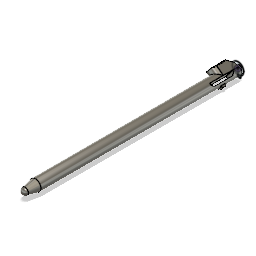
Nintendo 2DS Stylus v2 (Autodesk Fusion 360 design; units mm, degrees)
Autodesk Fusion 360 part; units mm, degrees
sketch "Sketch1" plane through (0, 0, 0) normal (0, 0, 1) x (1, 0, 0)
  circle A0 centre (0, 0) radius 2.45
  dimension "d1" = 4.9
  constraint coincident A0.centre origin
  measures "d1" diameter of A0
extrude "Extrude1" add sketch "Sketch1" along normal blind 94
sketch "Sketch2" plane through (0, 0, 0) normal (1, 0, 0) x (0, 0, -1)
  line L0 (0, 0) -> (0, -2.45)
  line L1 (0, -2.45) -> (-1, -2.45)
  line L2 (0, -2.45) -> (-3.2, -2.45)
  line L3 (-3.2, -2.45) -> (-3.2, 3.95)
  line L4 (-3.2, 3.95) -> (0, 3.95)
  line L5 (0, 3.95) -> (0, -2.45)
  line L6 (0, -2.45) -> (0, 1.95)
  line L7 (0, 1.95) -> (-1, 1.95)
  line L8 (0, -2.45) -> (-1, 1.95)
  line L9 (-1, 1.95) -> (-3.2, 3.95)
  line L10 (0, 0) -> (-3.2, 0)
  line L11 (-3.2, 3.95) -> (-10.3, 3.95)
  line L12 (-10.3, 3.95) -> (-3.2, 3.95)
  line L13 (-3.2, 3.95) -> (-3.2, 0)
  line L14 (-3.2, 0) -> (-10.3, 0)
  line L15 (-10.3, 0) -> (-10.3, 3.95)
  dimension "d4" = 2.45
  dimension "d5" = 1
  dimension "d8" = 3.2
  dimension "d9" = 6.4
  dimension "d10" = 4.4
  dimension "d11" = 1
  dimension "d14" = 7.1
  constraint coincident L0.start L10.start
  constraint vertical L0
  constraint horizontal L1
  constraint horizontal L2
  constraint vertical L3
  constraint horizontal L4
  constraint vertical L5
  constraint perpendicular L1 L6
  constraint perpendicular L6 L7
  constraint coincident L3 L10.end
  constraint perpendicular L3 L10
  constraint perpendicular L3 L11
  constraint horizontal L12
  constraint vertical L13
  constraint horizontal L14
  constraint vertical L15
  measures "d4" distance of L0.start L0.end
  measures "d5" distance of L0.end L1.end
  measures "d8" distance of L0.end L2.end
  measures "d9" distance of L0.end L4.end
  measures "d10" distance of L0.end L6.end
  measures "d11" distance of L6.end L7.end
  measures "d14" distance of L3.end L11.end
extrude "Extrude3" add sketch "Sketch2" along normal mid plane 4.9 contours L3 L8 L9 L10 L13 | L3 L11 L12 L13 L14 L15
extrude "Extrude2" cut sketch "Sketch2" along normal mid plane 12 contours L5 L6 L7 L8 L10 | L0 L5 L6 L8 L10 | L4 L5 L7 L9
sketch "Sketch3" plane through (0, 3.95, 0) normal (0, 1, 0) x (-1, 0, 0)
  line L0 (2.45, 10.3) -> (-2.45, 10.3)
  line L1 (-2.45, 10.3) -> (-2.45, 3.2)
  line L2 (-2.45, 3.2) -> (2.45, 3.2)
  line L3 (2.45, 3.2) -> (2.45, 10.3)
  circle A0 centre (0, 7.85) radius 2.45
  dimension "d17" = 4.9
  measures "d17" diameter of A0
extrude "Extrude4" cut sketch "Sketch3" against normal blind 4.1 contours L0 L3 A0 | L0 L1 A0
extrude "Extrude5" add 2 faces at (0.1162, 1.575, 10.3) (-0.1207, 1.5744, 10.3) along direction (0, 0, -1) blind 3.8
sketch "Sketch4" plane through (2.45, 0, 0) normal (1, 0, 0) x (0, 0, -1)
  line L0 (-7.85, 3.95) -> (-7.85, 0)
  line L1 (-7.85, 0) -> (-0.5568, 0)
  line L2 (-0.5568, 0) -> (-1, 1.95)
  line L3 (-1, 1.95) -> (-3.2, 3.95)
  line L4 (-3.2, 3.95) -> (-7.85, 3.95)
  line L5 (-3.2, 3.95) -> (-10.3, 3.95)
  line L6 (-10.3, 3.95) -> (-9.05, 3.95)
  line L7 (-9.05, 3.95) -> (-8.3, 3.95)
  line L8 (-8.3, 3.95) -> (-8.05, 3.95)
  line L9 (-8.05, 3.95) -> (-7.3, 3.95)
  line L10 (-7.3, 3.95) -> (-7.05, 3.95)
  line L11 (-7.05, 3.95) -> (-6.3, 3.95)
  line L12 (-6.3, 3.95) -> (-6.05, 3.95)
  line L13 (-6.05, 3.95) -> (-5.3, 3.95)
  line L14 (-8.675, 3.95) -> (-8.675, 3.45)
  line L15 (-9.05, 3.95) -> (-8.675, 3.45)
  line L16 (-8.675, 3.45) -> (-8.3, 3.95)
  line L17 (-7.675, 3.95) -> (-7.675, 3.45)
  line L18 (-6.675, 3.95) -> (-6.675, 3.45)
  line L19 (-5.675, 3.95) -> (-5.675, 3.45)
  line L20 (-8.05, 3.95) -> (-7.675, 3.45)
  line L21 (-7.675, 3.45) -> (-7.3, 3.95)
  line L22 (-7.05, 3.95) -> (-6.675, 3.45)
  line L23 (-6.3, 3.95) -> (-6.675, 3.45)
  line L24 (-6.05, 3.95) -> (-5.675, 3.45)
  line L25 (-5.675, 3.45) -> (-5.3, 3.95)
  line L26 (-5.3, 3.95) -> (-5.05, 3.95)
  line L27 (-5.05, 3.95) -> (-4.3, 3.95)
  line L28 (-4.675, 3.95) -> (-4.675, 3.45)
  line L29 (-5.05, 3.95) -> (-4.675, 3.45)
  line L30 (-4.675, 3.45) -> (-4.3, 3.95)
  dimension "d22" = 7.1
  dimension "d23" = 1.25
  dimension "d24" = 0.75
  dimension "d25" = 0.25
  dimension "d26" = 0.75
  dimension "d27" = 0.25
  dimension "d28" = 0.75
  dimension "d29" = 0.25
  dimension "d30" = 0.75
  dimension "d31" = 0.5
  dimension "d32" = 0.5
  dimension "d33" = 0.5
  dimension "d34" = 0.5
  dimension "d35" = 0.25
  dimension "d36" = 0.75
  dimension "d37" = 0.5
  constraint coincident L3.end L4.start
  constraint perpendicular L0 L5
  constraint parallel L5 L6
  constraint parallel L5 L7
  constraint parallel L5 L8
  constraint perpendicular L0 L9
  constraint parallel L4 L10
  constraint parallel L5 L11
  constraint parallel L5 L12
  constraint parallel L5 L13
  constraint midpoint L7 L14.start
  constraint perpendicular L7 L14
  constraint midpoint L9 L17.start
  constraint perpendicular L5 L17
  constraint midpoint L11 L18.start
  constraint perpendicular L5 L18
  constraint midpoint L13 L19.start
  constraint perpendicular L13 L19
  constraint coincident L4 L26.end
  constraint parallel L5 L27
  constraint midpoint L27 L28.start
  constraint perpendicular L5 L28
  measures "d22" distance of L3.end L5.end
  measures "d23" distance of L5.end L6.end
  measures "d24" distance of L6.end L7.end
  measures "d25" distance of L7.end L8.end
  measures "d26" distance of L8.end L9.end
  measures "d27" distance of L9.end L10.end
  measures "d28" distance of L10.end L11.end
  measures "d29" distance of L11.end L12.end
  measures "d30" distance of L12.end L13.end
  measures "d31" distance of L14.start L14.end
  measures "d32" distance of L17.start L17.end
  measures "d33" distance of L18.start L18.end
  measures "d34" distance of L19.start L19.end
  measures "d35" distance of L13.end L26.end
  measures "d36" distance of L26.end L27.end
  measures "d37" distance of L28.start L28.end
extrude "Extrude6" cut sketch "Sketch4" against normal blind 8.9 contours L0 L4 L5 L9 L17 L20 | L0 L5 L9 L20 | L4 L5 L9 L17 L21 | L4 L5 L11 L18 L22 | L4 L5 L11 L18 L23 | L4 L5 L27 L28 L30 | L4 L5 L13 L19 L24 | L4 L5 L27 L28 L29 | L4 L5 L13 L19 L25 | L5 L7 L14 L16 | L5 L7 L14 L15
sketch "Sketch5" plane through (0, 0, 0) normal (1, 0, 0) x (0, 0, -1)
  line L0 (0, 0) -> (0, -2.45)
  line L1 (0, -2.45) -> (-9.8, -2.45)
  line L2 (-9.8, -2.45) -> (-7.8, -2.45)
  ellipse E0 centre (-8.8, -2.45) end of major axis (-7.8, -2.45) minor radius 0.625
  line L3 (-9.8, -2.45) -> (-7.8, -2.45) construction
  line L4 (-8.8, -3.075) -> (-8.8, -1.825) construction
  line L5 (0, 0) -> (-8.8, 0)
  line L6 (-8.8, -2.45) -> (-8.8, -1.45)
  line L7 (-8.8, 0) -> (-3.8, 0)
  line L8 (-3.8, 1.45) -> (-13.8, 1.45)
  line L9 (-13.8, -1.45) -> (-3.8, -1.45)
  line L10 (-3.8, 0) -> (-13.8, 0) construction
  line L11 (-8.8, 0) -> (-15.25, 0)
  line L12 (-5.25, 1.45) -> (-12.35, 1.45)
  arc A0 (-12.35, 1.45) -> (-12.35, -1.45) centre (-12.35, 0) ccw
  line L13 (-12.35, -1.45) -> (-5.25, -1.45)
  arc A1 (-5.25, -1.45) -> (-5.25, 1.45) centre (-5.25, 0) ccw
  line L14 (-3.8, 0) -> (-13.8, 0) construction
  dimension "d40" = 2.45
  dimension "d41" = 9.8
  dimension "d42" = 2
  dimension "d43" = 1.25
  dimension "d44" = 1
  dimension "d45" = 5
  constraint coincident L0.start L5.start
  constraint vertical L0
  constraint perpendicular L0 L1
  constraint parallel L1 L2
  constraint midpoint L2 E0.centre
  constraint coincident L1.end E0
  constraint coincident E0 L4.start
  constraint coincident E0 L4.end
  constraint perpendicular L4 L5
  constraint coincident E0.centre L6.start
  constraint perpendicular L3 L6
  constraint parallel L5 L7
  constraint parallel L8 L9
  constraint parallel L5 L10
  constraint coincident L7.end L10.start
  constraint tangent L12 A0
  constraint tangent A0 L13
  constraint parallel L12 L13
  constraint tangent L13 A1
  constraint tangent L12 A1
  constraint midpoint A1 L7.end
  constraint midpoint A0 L10.end
  constraint coincident L10.end L14.end
  constraint parallel L11 L14
  measures "d40" distance of L0.start L0.end
  measures "d41" distance of L0.end L1.end
  measures "d42" distance of L1.end L2.end
  measures "d44" distance of E0.centre L6.end
  measures "d45" distance of L5.end L7.end
extrude "Extrude7" cut sketch "Sketch5" along normal mid plane 11 contours L5 L7 L9 L11 A0 L13 A1
extrude "Extrude8" add sketch "Sketch5" along normal mid plane 2 contours L1 L2 E0 | L1 L2 E0 L6 | L1 L2 E0 L6
sketch "Sketch6" plane through (0, 0, 94) normal (0, 0, 1) x (1, 0, 0)
  circle A0 centre (0, 0) radius 2.45
  circle A1 centre (0, 0) radius 1.5
  dimension "d50" = 3
  constraint coincident A0.centre A1.centre
  measures "d50" diameter of A1
extrude "Extrude9" cut sketch "Sketch6" against normal blind 6
fillet "Fillet1" radius 1.5 1 edges at (-1.3985, -0.5424, 94)
chamfer "Chamfer1" distance 4.5 distance2 0.95 1 edges at (-1.3985, -0.5424, 88) measured on face at (1.4981, -0.0748, 89.5)
move_face "OffsetFaces1" offset -0.5 2 faces at (0.8167, 0.65, 0.7045) (-0.8167, 2.6167, 1.7333)
sketch "Sketch7" plane through (0, 0, 0) normal (0, 0, 1) x (1, 0, 0)
  circle A0 centre (0, 0) radius 2.45
  line L0 (0, 0) -> (0, -3.075)
  line L1 (0, -3.075) -> (1, -3.075)
  line L2 (1, -3.075) -> (1, -2.2366)
  line L3 (1, -2.2366) -> (0, -2.2366)
  line L4 (0, -2.2366) -> (0, -3.075)
  line L5 (1, -3.075) -> (0.75, -3.075)
  line L6 (0.75, -3.075) -> (1.9563, -1.4749)
  dimension "d57" = 4.9
  dimension "d58" = 3.075
  dimension "d59" = 1
  dimension "d60" = 0.25
  constraint coincident A0.centre L0.start
  constraint vertical L0
  constraint horizontal L1
  constraint vertical L2
  constraint horizontal L3
  constraint vertical L4
  constraint coincident A0 L2.end
  constraint perpendicular L2 L5
  constraint coincident A0 L6.end
  constraint tangent A0 L6
  measures "d57" diameter of A0
  measures "d58" distance of A0.centre L0.end
  measures "d59" distance of L0.end L1.end
  measures "d60" distance of L1.end L5.end
move_body "Move1" bodies 1 to x (0.601815, 0.798636, 0) y (-0.798636, 0.601815, 0) z (0, 0, 1) at (0, 0, 0)
equation "d4 = ( 4.9 / 2 ) * 1 mm"
equation "d15 = ( 4.9 / 2 ) * 1 mm"
equation "d40 = ( 4.9 / 2 ) * 1 mm"
equation "d56 = ( ( 4.9 - 3 ) / 2 ) * 1 mm"
equation "d58 = ( ( 4.9 / 2 ) * 1 mm ) + ( ( 1.25 / 2 ) * 1 mm )"
named bodies: "2DS Stylus"
